Autodesk Inventor part; units mm, degrees
(part 2 of 2)
sketch "Sketch64" plane through (-85, 0, -85) normal (1, 0, 0) x (0, 0, -1)
  line L0 (-135, 92.7054) -> (-35, 92.7054)
  line L1 (-35, 92.7054) -> (-35, 82.7054)
  line L2 (-35, 82.7054) -> (-135, 82.7054)
  line L3 (-135, 82.7054) -> (-135, 92.7054)
  line L4 (-135, 227.7054) -> (-35, 227.7054)
  line L5 (-35, 227.7054) -> (-35, 217.7054)
  line L6 (-35, 217.7054) -> (-135, 217.7054)
  line L7 (-135, 217.7054) -> (-135, 227.7054)
  line L8 (0, 564.1154) -> (-170, 564.1154) projected
  line L9 (0, 0) -> (-170, 0) projected
  line L10 (-130, 504.1154) -> (-40, 504.1154)
  line L11 (-40, 504.1154) -> (-40, 524.1154)
  line L12 (-40, 524.1154) -> (-130, 524.1154)
  line L13 (-130, 524.1154) -> (-130, 504.1154)
  line L14 (-130, 509.1154) -> (-40, 509.1154)
  line L15 (-40, 509.1154) -> (-40, 519.1154)
  line L16 (-40, 519.1154) -> (-130, 519.1154)
  line L17 (-130, 519.1154) -> (-130, 509.1154)
  line L18 (-135, 60) -> (-35, 60)
  line L19 (-35, 60) -> (-35, 65)
  line L20 (-35, 65) -> (-135, 65)
  line L21 (-135, 65) -> (-135, 60)
  point P0 (-85, 0)
  point P1 (-85, 227.7054)
  point P2 (-85, 0)
  point P3 (-85, 564.1154)
  point P4 (-85, 564.1154)
  point P5 (-85, 564.1154)
  point P6 (-85, 524.1154)
  point P7 (-130, 514.1154)
  point P8 (-35, 62.5)
  dimension "d723" = 336.41
  dimension "d724" = 10
  dimension "d725" = 100
  dimension "d726" = 125
  dimension "d727" = 10
  dimension "d762" = 90
  dimension "d763" = 20
  dimension "d764" = 40
  dimension "d765" = 10
  dimension "d791" = 60
  dimension "d792" = 5
  constraints: 40 end point, 10 parallel, 9 midpoint, 6 point on line, 5 horizontal, 5 perpendicular, 2 vertical alignment
  measures "d723" distance between parallel lines of L4 L8
  measures "d724" distance of L4.end L5.end
  measures "d725" distance of L4.start L4.end
  measures "d726" distance between parallel lines of L0 L6
  measures "d727" distance of L0.end L1.end
  measures "d762" distance of L11.end L12.end
  measures "d763" distance of L10.end L11.end
  measures "d764" distance between parallel lines of L12 L8
  measures "d765" distance between parallel lines of L14 L16
  measures "d791" distance between parallel lines of L18 L9
  measures "d792" distance of L20.end L18.start
extrude "Extrusion37" add sketch "Sketch64" along normal blind 5 contours L0 L1 L2 L3 | L4 L5 L6 L7 | L21 L20 L19 L18 bodies 13
extrude "Extrusion39" add sketch "Sketch64" along normal blind 5 contours L13 L14 L11 L10 | L13 L16 L11 L14 | L13 L12 L11 L16 bodies 13
extrude "Extrusion40" cut sketch "Sketch64" against normal blind 3 from surface at 5 contours L13 L16 L11 L14 bodies 13
sketch "Sketch67" plane through (-83, 509.1154, 45) normal (1, 0, 0) x (0, 0, -1)
  line L0 (0, 10) -> (0, 0) construction
  line L1 (0, 5) -> (90, 5) construction
  line L2 (90, 0) -> (90, 10) construction
  point P0 (45, -509.1154)
  point P1 (15, 5)
  point P2 (75, 5)
  dimension "d778" = 60
  dimension "d779" = 15
  constraints: 2 end point, 2 midpoint, 2 point on line
  measures "d778" distance of point (75, 5) point (15, 5)
  measures "d779" distance from line of L0 point (15, 5)
hole "Hole31" at (-83, 514.1154, 30) at (-83, 514.1154, -30) direction (-1, 0, 0) diameter 2.459 depth 5 tip angle 118 bodies 13
sketch "Sketch69" plane through (-80, 0, -85) normal (1, 0, 0) x (0, 0, -1)
  line L0 (-135, 92.7054) -> (-135, 82.7054) construction
  line L1 (-135, 87.7054) -> (-35, 87.7054) construction
  line L2 (-35, 92.7054) -> (-35, 82.7054) construction
  line L3 (-135, 217.7054) -> (-135, 227.7054) construction
  line L4 (-135, 222.7054) -> (-35, 222.7054) construction
  line L5 (-35, 227.7054) -> (-35, 217.7054) construction
  point P0 (-85, 0)
  point P1 (-110, 87.7054)
  point P2 (-60, 87.7054)
  point P3 (-110, 222.7054)
  point P4 (-60, 222.7054)
  point P5 (-85, 87.7054)
  point P6 (-85, 222.7054)
  dimension "d800" = 25
  dimension "d802" = 25
  dimension "d803" = 25
  dimension "d804" = 25
  dimension "d805" = 25
  dimension "d806" = 25
  constraints: 6 midpoint, 4 end point, 4 point on line
  measures "d800" distance from line of L0 point (-110, 87.705)
  measures "d802" distance from line of L3 point (-110, 222.705)
  measures "d803" distance from line of L5 point (-60, 222.705)
  measures "d804" distance of point (-110, 87.705) point (-85, 87.705)
  measures "d805" distance of point (-60, 87.705) point (-85, 87.705)
  measures "d806" distance of point (-60, 222.705) point (-85, 222.705)
hole "Hole33" at (-80, 87.7054, 25) at (-80, 87.7054, -25) at (-80, 222.7054, 25) at (-80, 222.7054, -25) at (-80, 87.7054, 0) at (-80, 222.7054, 0) direction (-1, 0, 0) diameter 2.459 depth 5 tip angle 118 bodies 13
body "Solid3"
body "Solid12"
body "Solid25"
body "Solid26"
body "Solid27"
body "Solid29"
body "Solid18"
body "Solid19"
body "Solid20"
body "Solid23"
